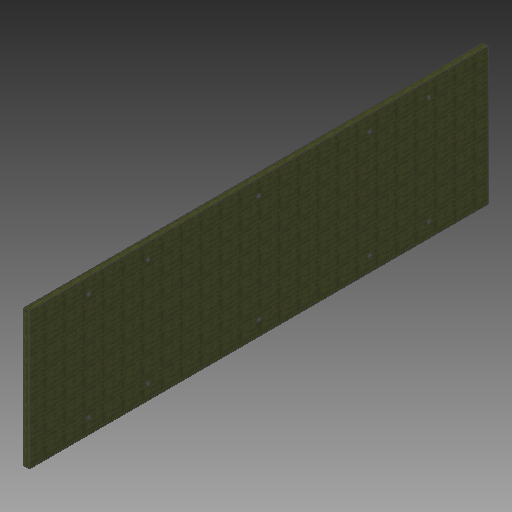
# Autodesk Inventor part: 1212_Flat Connector_V1
Saved by Autodesk Inventor 2020 (Build 240168000, 168)
## iProperties
Created: 2017-06-14
Part Number: 1212_Flat Connector_V1
Material: GFRP
Document SubType Name: Modeling
Designer: MPI
Density: 1.75 g/cm^3
Appearance: Smooth - Light Gray
Mass: 384.75 g
Surface Area: 976.915 cm^2
Volume: 219.857 cm^3
Author: MPI
Autodesk Inventor part; units mm, degrees
ref_plane "YZ Plane" through (0, 0, 0) normal (1, 0, 0) x (0, 1, 0)
ref_plane "XZ Plane" through (0, 0, 0) normal (0, 1, 0) x (-1, 0, 0)
ref_plane "XY Plane" through (0, 0, 0) normal (0, 0, 1) x (1, 0, 0)
sketch "Sketch3" plane through (0, 0, 0) normal (0, 0, 1) x (1, 0, 0)
  line L0 (-58.7375, -58.7375) -> (58.7375, -58.7375)
  line L1 (58.7375, -58.7375) -> (58.7375, 58.7375)
  line L2 (58.7375, 58.7375) -> (-58.7375, 58.7375)
  line L3 (-58.7375, 58.7375) -> (-58.7375, -58.7375)
  line L4 (-58.7375, -58.7375) -> (58.7375, 58.7375) construction
  line L5 (58.7375, -58.7375) -> (-58.7375, 58.7375) construction
  line L6 (63.5, -58.7375) -> (63.5, 58.7375)
  line L7 (-63.5, 58.7375) -> (-63.5, -58.7375)
  line L8 (-58.7375, 58.7375) -> (-63.5, 58.7375)
  line L9 (58.7375, 58.7375) -> (63.5, 58.7375)
  line L10 (58.7375, -58.7375) -> (63.5, -58.7375)
  line L11 (-58.7375, -58.7375) -> (-63.5, -58.7375)
  point P0 (0, 0)
  dimension "d28" = 117.475
  dimension "d29" = 117.475
  dimension "d30" = 4.7625
  dimension "d40" = 4.7625
  constraints: 24 end point, 4 perpendicular, 3 parallel, 2 midpoint, 1 horizontal, 1 point on line
  measures "d28" distance of L2.end L1.end
  measures "d29" distance of L1.end L0.end
  measures "d30" distance between parallel lines of L3 L7
  measures "d40" distance between parallel lines of L6 L1
extrude "Extrusion3" add sketch "Sketch3" along normal mid plane 393.7 contours L1 L9 L6 L10
sketch "Sketch7" plane through (58.7375, -58.7375, 196.85) normal (-1, 0, 0) x (0, 0, 1)
  line L0 (-393.7, 0) -> (0, 0) projected
  line L1 (0, 117.475) -> (0, 0) projected
  line L2 (0, 117.475) -> (-393.7, 117.475) projected
  line L3 (-393.7, 0) -> (-393.7, 117.475) projected
  line L4 (-393.7, 117.475) -> (-393.7, 0) projected
  line L5 (-393.7, 104.775) -> (0, 104.775)
  point P0 (-196.85, 58.7375)
  point P1 (-342.9, 104.775)
  point P2 (-196.85, 104.775)
  point P3 (-292.1, 104.775)
  point P4 (-50.8, 104.775)
  point P5 (-101.6, 104.775)
  dimension "d47" = 12.7
  dimension "d48" = 50.8
  dimension "d49" = 50.8
  dimension "d50" = 50.8
  dimension "d51" = 50.8
  constraints: 6 point on line, 2 end point, 1 midpoint, 1 perpendicular
  measures "d47" distance between parallel lines of L2 L5
  measures "d48" distance from line of L3 point (-342.9, 104.775)
  measures "d49" distance of point (-342.9, 104.775) point (-292.1, 104.775)
  measures "d50" distance of L5.end point (-50.8, 104.775)
  measures "d51" distance of point (-50.8, 104.775) point (-101.6, 104.775)
hole "Hole2" at (58.7375, 46.0375, -146.05) at (58.7375, 46.0375, 0) at (58.7375, 46.0375, -95.25) at (58.7375, 46.0375, 146.05) at (58.7375, 46.0375, 95.25) direction (1, 0, 0) diameter 3.302 depth 12.446 tip angle 118 thread size "8-32 UNC" class "2B" standard "ANSI Unified Screw Threads"
mirror "Mirror7" about plane through (0, 0, 0) normal (0, 1, 0) of "Hole2"
equation "\"d40\" = d30"
equation "\"d49\" = d48"
equation "\"d50\" = d48"
equation "\"d51\" = d50"
body "Solid1"
body "Solid2"
